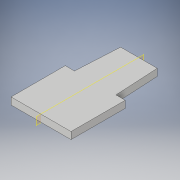
# Autodesk Inventor part: Motor Mount
Saved by Autodesk Inventor 2018 (Build 220112000, 112)
## iProperties
Created: 2018-08-09
Part Number: Motor Mount
Material: Generic
Document SubType Name: Modeling
Designer: Michael Gunderman
Density: 1 g/cm^3
Appearance: Default
Author: Michael Gunderman
Autodesk Inventor part; units mm, degrees
ref_plane "YZ Plane" through (0, 0, 0) normal (1, 0, 0) x (0, 1, 0)
ref_plane "XZ Plane" through (0, 0, 0) normal (0, 1, 0) x (-1, 0, 0)
ref_plane "XY Plane" through (0, 0, 0) normal (0, 0, 1) x (1, 0, 0)
sketch "Sketch1" plane through (0, 0, 0) normal (0, 1, 0) x (-1, 0, 0)
  line L0 (0, 0) -> (-30, 0)
  line L1 (-30, 0) -> (-30, -98)
  line L2 (0, 0) -> (0, -54.2421)
  line L3 (0, -54.2421) -> (-9.2274, -54.2421)
  line L4 (-9.2274, -54.2421) -> (-11.6739, -98)
  line L5 (-11.6739, -98) -> (-30, -98)
  line L6 (-60, 0) -> (-30, 0)
  line L7 (-60, 0) -> (-60, -54.2421)
  line L8 (-60, -54.2421) -> (-50.7726, -54.2421)
  line L9 (-50.7726, -54.2421) -> (-48.3261, -98)
  line L10 (-48.3261, -98) -> (-30, -98)
  dimension "d4" = 98
  dimension "d7" = 30
  constraints: 22 end point, 4 symmetric about line, 2 vertical, 1 horizontal, 1 parallel, 1 perpendicular
  measures "d4" distance of L0.end L1.end
  measures "d7" distance between parallel lines of L1 L2
extrude "Extrusion2" add sketch "Sketch1" along normal blind 7
ref_plane "Work Plane1" through (30, 0, 0) normal (1, 0, 0) x (0, 0, -1)
body "Solid2"
